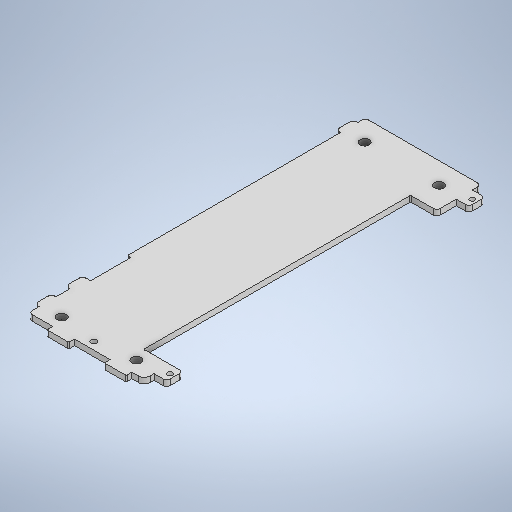
# Autodesk Inventor part: 21-30-220-B2
Saved by Autodesk Inventor 2025.2 (Build 292293000, 293)
## iProperties
Created: 2024-11-14
Part Number: 21-30-220-B2
Material: Generic
Document SubType Name: Sheet Metal
Designer: Zvonko.Gabric
Density: 1 g/cm^3
Appearance: Default
Sheet Metal Rule: Default
Description: Center panel,
Author: Zvonko.Gabric
Autodesk Inventor part; units mm, degrees
ref_plane "YZ Plane" through (0, 0, 0) normal (1, 0, 0) x (0, 1, 0)
ref_plane "XZ Plane" through (0, 0, 0) normal (0, 1, 0) x (-1, 0, 0)
ref_plane "XY Plane" through (0, 0, 0) normal (0, 0, 1) x (1, 0, 0)
sketch "Sketch1" plane through (0, 0, 0) normal (0, 1, 0) x (-1, 0, 0)
  line L0 (0, 0) -> (31, 0)
  line L1 (31, 0) -> (31, 4)
  line L2 (32, 5) -> (49, 5)
  line L3 (50, 4) -> (50, 0)
  line L4 (50, 0) -> (68, 0)
  line L5 (68, -52) -> (68, -85)
  line L6 (69, -86) -> (70, -86)
  line L7 (71, -87) -> (71, -272.1)
  line L8 (71, -272.1) -> (72.1718, -272.1)
  line L9 (72.8789, -272.3929) -> (74.7071, -274.2211)
  line L10 (75, -274.9282) -> (75, -284.1718)
  line L11 (74.7071, -284.8789) -> (72.8789, -286.7071)
  line L12 (72.1718, -287) -> (71, -287)
  line L13 (71, -287) -> (71, -293.6)
  line L14 (71, -293.6) -> (-26.8, -293.6)
  line L15 (-29.8, -290.6) -> (-29.8, -286)
  line L16 (0, 0) -> (0, 4)
  line L17 (-1, 5) -> (-18, 5)
  line L18 (-19, 4) -> (-19, 0)
  line L19 (-19, 0) -> (-24.8, 0)
  line L20 (-29.8, -5) -> (-29.8, -8.5)
  line L21 (-29.8, -8.5) -> (-37.8, -8.5)
  line L22 (-40.8, -11.5) -> (-40.8, -19.5)
  line L23 (-37.8, -22.5) -> (-7.9, -22.5)
  line L24 (-6.9, -23.5) -> (-6.9, -254)
  line L25 (-7.9, -255) -> (-26.8, -255)
  line L26 (-29.8, -258) -> (-29.8, -272)
  line L27 (-29.8, -272) -> (-37.8, -272)
  line L28 (-40.8, -275) -> (-40.8, -283)
  line L29 (-37.8, -286) -> (-29.8, -286)
  circle A0 centre (53.1, -11) radius 4
  circle A1 centre (-11.9, -11) radius 4
  circle A2 centre (53.1, -275) radius 4
  circle A3 centre (-11.9, -275) radius 4
  line L30 (69, -51) -> (70, -51)
  arc A4 (-18, 5) -> (-19, 4) centre (-18, 4) ccw
  arc A5 (0, 4) -> (-1, 5) centre (-1, 4) ccw
  arc A6 (32, 5) -> (31, 4) centre (32, 4) ccw
  arc A7 (50, 4) -> (49, 5) centre (49, 4) ccw
  arc A8 (-24.8, 0) -> (-29.8, -5) centre (-24.8, -5) ccw
  arc A9 (-7.9, -255) -> (-6.9, -254) centre (-7.9, -254) ccw
  arc A10 (-26.8, -255) -> (-29.8, -258) centre (-26.8, -258) ccw
  arc A11 (-37.8, -272) -> (-40.8, -275) centre (-37.8, -275) ccw
  arc A12 (-40.8, -283) -> (-37.8, -286) centre (-37.8, -283) ccw
  arc A13 (-40.8, -19.5) -> (-37.8, -22.5) centre (-37.8, -19.5) ccw
  arc A14 (-37.8, -8.5) -> (-40.8, -11.5) centre (-37.8, -11.5) ccw
  arc A15 (72.8789, -272.3929) -> (72.1718, -272.1) centre (72.1718, -273.1) ccw
  arc A16 (75, -274.9282) -> (74.7071, -274.2211) centre (74, -274.9282) ccw
  arc A17 (74.7071, -284.8789) -> (75, -284.1718) centre (74, -284.1718) ccw
  arc A18 (72.1718, -287) -> (72.8789, -286.7071) centre (72.1718, -286) ccw
  line L31 (71, -9.1) -> (72.1718, -9.1)
  line L32 (72.8789, -9.3929) -> (74.7071, -11.2211)
  line L33 (75, -11.9282) -> (75, -21.1718)
  line L34 (74.7071, -21.8789) -> (72.8789, -23.7071)
  line L35 (72.1718, -24) -> (71, -24)
  arc A19 (72.8789, -9.3929) -> (72.1718, -9.1) centre (72.1718, -10.1) ccw
  arc A20 (75, -11.9282) -> (74.7071, -11.2211) centre (74, -11.9282) ccw
  arc A21 (74.7071, -21.8789) -> (75, -21.1718) centre (74, -21.1718) ccw
  arc A22 (72.1718, -24) -> (72.8789, -23.7071) centre (72.1718, -23) ccw
  line L36 (71, -36.1) -> (72.1718, -36.1)
  line L37 (72.8789, -36.3929) -> (74.7071, -38.2211)
  line L38 (75, -38.9282) -> (75, -48.1718)
  line L39 (74.7071, -48.8789) -> (72.8789, -50.7071)
  line L40 (72.1718, -51) -> (71, -51)
  arc A23 (72.8789, -36.3929) -> (72.1718, -36.1) centre (72.1718, -37.1) ccw
  arc A24 (75, -38.9282) -> (74.7071, -38.2211) centre (74, -38.9282) ccw
  arc A25 (74.7071, -48.8789) -> (75, -48.1718) centre (74, -48.1718) ccw
  arc A26 (72.1718, -51) -> (72.8789, -50.7071) centre (72.1718, -50) ccw
  line L41 (71, -9.1) -> (71, -3)
  line L42 (71, -24) -> (71, -36.1)
  arc A27 (69, -51) -> (68, -52) centre (69, -52) ccw
  arc A28 (68, -85) -> (69, -86) centre (69, -85) ccw
  arc A29 (71, -87) -> (70, -86) centre (70, -87) ccw
  line L43 (71, -51) -> (70, -51)
  arc A30 (71, -3) -> (68, 0) centre (68, -3) ccw
  arc A31 (-6.9, -23.5) -> (-7.9, -22.5) centre (-7.9, -23.5) ccw
  arc A32 (-29.8, -290.6) -> (-26.8, -293.6) centre (-26.8, -290.6) ccw
  circle A33 centre (-36.8, -15.5) radius 2.15
  circle A34 centre (-36.8, -279) radius 2.15
  circle A35 centre (20.6, -6.5) radius 2.5
  point P0 (31, 5)
  point P1 (50, 5)
  point P2 (71, 0)
  point P3 (68, -86)
  point P4 (71, -86)
  point P5 (72.586, -272.1)
  point P6 (72.586, -287)
  point P7 (0, 5)
  point P8 (59, 0)
  point P9 (50, 2)
  point P10 (71, -5)
  point P11 (-22.85, -22.5)
  point P12 (-33.8, -8.5)
  point P13 (71.5859, -287)
  point P14 (71.8793, -10)
  point P15 (69.5, -51)
  point P16 (-21.9, 0)
  point P17 (71.5859, -24)
  point P18 (71.5859, -51)
  point P19 (69.5, -86)
  point P20 (-29.8, -6.75)
  point P21 (40.5, 5)
  dimension "d0" = 90
  dimension "d1" = 31
  dimension "d3" = 19
  dimension "d4" = 19
  dimension "d8" = 14
  dimension "d10" = 0
  dimension "d11" = 8
  dimension "d12" = 11
  dimension "d13" = 8
  dimension "d14" = 65
  dimension "d15" = 8
  dimension "d16" = 8
  dimension "d17" = 264
  dimension "d18" = 264
  dimension "d21" = 3
  dimension "d24" = 51
  dimension "d25" = 5
  dimension "d26" = 5
  dimension "d27" = 1
  dimension "d28" = 5
  dimension "d30" = 77.9
  dimension "d32" = 1
  dimension "d33" = 3
  dimension "d34" = 17
  dimension "d35" = 14
  dimension "d36" = 11
  dimension "d37" = 3
  dimension "d38" = 22.5
  dimension "d39" = 33.9
  dimension "d40" = 3
  dimension "d41" = 11
  dimension "d42" = 4
  dimension "d43" = 14.9
  dimension "d44" = 6.6
  dimension "d45" = 1.586
  dimension "d46" = 135
  dimension "d47" = 1.586
  dimension "d48" = 135
  dimension "d49" = 1
  dimension "d50" = 14.9
  dimension "d51" = 135
  dimension "d52" = 135
  dimension "d53" = 1
  dimension "d54" = 14.9
  dimension "d55" = 135
  dimension "d56" = 135
  dimension "d57" = 1
  dimension "d58" = 9.1
  dimension "d59" = 12.1
  dimension "d61" = 1
  dimension "d62" = 35
  dimension "d63" = 100.8
  dimension "d64" = 38.6
  dimension "d67" = 3
  dimension "d68" = 1
  dimension "d69" = 3
  dimension "d70" = 232.5
  dimension "d71" = 27.5
  dimension "d74" = 293.6
  dimension "d75" = 185.1
  dimension "d76" = 4.3
  dimension "d77" = 4
  dimension "d78" = 7
  dimension "d79" = 4
  constraints: 88 end point, 58 point on circle, 58 tangent, 36 centre point, 21 perpendicular, 20 point on line, 16 equal radius, 12 midpoint, 4 vertical, 3 horizontal, 1 parallel
  measures "d0" angle of L2 L1
  measures "d1" distance of L0.start L0.end
  measures "d3" distance between parallel lines of L16 L18
  measures "d4" distance of point (31, 5) point (50, 5)
  measures "d8" distance from line of point (-33.8, -8.5) L23
  measures "d10" distance from line of L0.start L19
  measures "d11" diameter of A0
  measures "d12" distance from line of L4 A0.centre
  measures "d13" diameter of A1
  measures "d14" distance of A0.centre A1.centre
  measures "d15" diameter of A2
  measures "d16" diameter of A3
  measures "d17" distance of A2.centre A0.centre
  measures "d18" distance of A1.centre A3.centre
  measures "d21" distance of point (68, -86) point (71, -86)
  measures "d24" distance from line of L4 point (69.5, -51)
  measures "d25" distance of point (50, 5) L3.end
  measures "d26" distance of L0.start point (0, 5)
  measures "d27" radius of A4
  measures "d28" radius of A8
  measures "d30" distance between parallel lines of L7 L24
  measures "d32" radius of A9
  measures "d33" radius of A10
  measures "d34" distance between parallel lines of L27 L25
  measures "d35" distance between parallel lines of L27 L29
  measures "d36" distance between parallel lines of L15 L28
  measures "d37" radius of A11
  measures "d38" distance between parallel lines of L19 L23
  measures "d39" distance between parallel lines of L24 L22
  measures "d40" radius of A13
  measures "d41" distance between parallel lines of L20 L22
  measures "d42" distance between parallel lines of L7 L10
  measures "d43" distance between parallel lines of L12 L8
  measures "d44" distance of L12.end L13.end
  measures "d45" distance of L7.end point (72.586, -272.1)
  measures "d46" angle of L9 L8
  measures "d47" distance of point (72.586, -287) L12.end
  measures "d48" angle of L12 L11
  measures "d49" radius of A15
  measures "d50" distance between parallel lines of L35 L31
  measures "d51" angle of L32 L31
  measures "d52" angle of L35 L34
  measures "d53" radius of A19
  measures "d54" distance between parallel lines of L40 L36
  measures "d55" angle of L37 L36
  measures "d56" angle of L40 L39
  measures "d57" radius of A23
  measures "d58" distance of L31.start point (71, 0)
  measures "d59" distance of L35.end L36.start
  measures "d61" radius of A27
  measures "d62" distance from line of point (69.5, -86) L30
  measures "d63" distance from line of point (-29.8, -6.75) L41
  measures "d64" distance between parallel lines of L14 L25
  measures "d67" radius of A30
  measures "d68" radius of A31
  measures "d69" radius of A32
  measures "d70" distance between parallel lines of L23 L25
  measures "d71" distance between parallel lines of L17 L23
  measures "d74" distance between parallel lines of L4 L14
  measures "d75" distance of L7.start L7.end
  measures "d76" diameter of A33
  measures "d77" distance from line of L22 A33.centre
  measures "d78" distance from line of L21 A33.centre
  measures "d79" distance from line of L28 A34.centre
extrude "Extrusion1" add sketch "Sketch1" along normal blind 5 contours L0 L1 A6 L2 A7 L3 L4 A30 L41 L31 A19 L32 A20 L33 A21 L34 A22 L35 L42 L36 A23 L37 A24 L38 A25 L39 A26 L40 L43 L30 A27 L5 A28 L6 A29 L7 L8 A15 L9 A16 L10 A17 L11 A18 L12 L13 L14 A32 L15 L29 A12 L28 A11 L27 L26 A10 L25 A9 L24 A31 L23 A13 L22 A14 L21 L20 A8 L19 L18 A4 L17 A5 L16 | A33 | A34 | A35
extrude "Extrusion2" cut sketch "Sketch1" along normal blind 5 contours A33 | A34 | A35
fillet "Fillet1" radius 3 1 edges at (-71, 2.5, -293.6)
thread "Thread1" size "M8x1.25" class "6H" standard "ANSI Metric M Profile" length 5
thread "Thread2" size "M8x1.25" class "6H" standard "ANSI Metric M Profile" length 5
thread "Thread3" size "M8x1.25" class "6H" standard "ANSI Metric M Profile" length 5
thread "Thread4" size "M8x1.25" class "6H" standard "ANSI Metric M Profile" length 5
body "Solid1"
